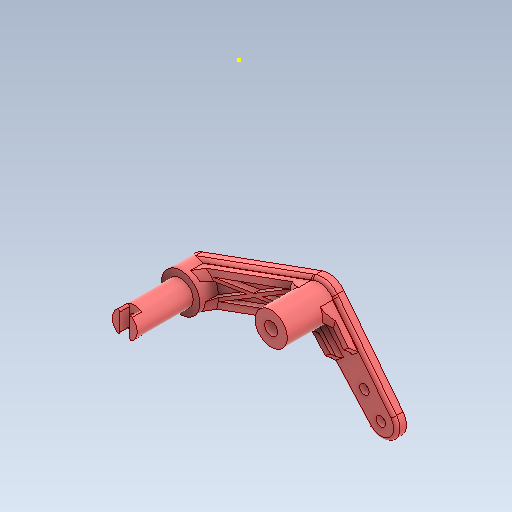
# Autodesk Inventor part: РычагОпорного
Saved by Autodesk Inventor 2020 (Build 240168000, 168)
## iProperties
Created: 2021-03-04
Part Number: РычагОпорного
Material: Пластик АБС
Document SubType Name: Modeling
Designer: I_Love_U_Bogdan
Density: 1.06 g/cm^3
Appearance: Гладкий — красный
Author: I_Love_U_Bogdan
Autodesk Inventor part; units mm, degrees
ref_plane "YZ Plane" through (0, 0, 0) normal (1, 0, 0) x (0, 1, 0)
ref_plane "XZ Plane" through (0, 0, 0) normal (0, 1, 0) x (-1, 0, 0)
ref_plane "XY Plane" through (0, 0, 0) normal (0, 0, 1) x (1, 0, 0)
sketch "Эскиз1" plane through (0, 0, 0) normal (0, 0, 1) x (1, 0, 0)
  arc A0 (12.888162, -136.868324) -> (8.919216, -139.740164) centre (9.43816, -136.27885) ccw
  line L0 (65.630259, -98.70533) -> (12.888162, -136.868324)
  arc A1 (69.599205, -95.83349) -> (65.630259, -98.70533) centre (66.149202, -95.244015) ccw
  line L1 (72.61468, -93.65156) -> (69.599205, -95.83349)
  line L2 (74.525657, -81.736041) -> (72.61468, -93.65156)
  arc A2 (78.84072, -74.295729) -> (74.525657, -81.736041) centre (86.374247, -83.636285) ccw
  arc A3 (78.84072, -74.295729) -> (86.631259, -62.29521) centre (64.401461, -56.392998) ccw
  line L3 (16.222884, -53.884997) -> (16.238465, -53.891971)
  line L4 (2.811002, -47.882385) -> (16.222884, -53.884997)
  line L5 (-128.593437, -142.96368) -> (2.811002, -47.882385)
  arc A4 (-128.593437, -142.96368) -> (-138.339207, -175.63158) centre (-112.179504, -165.648097) ccw
  line L6 (-101.16011, -190.130237) -> (-15.58744, -157.472629)
  line L7 (8.919216, -139.740164) -> (-15.58744, -157.472629)
  circle A5 centre (64.401461, -56.392998) radius 9
  circle A6 centre (25.088911, -52.746159) radius 2.05
  circle A7 centre (25.088911, -52.746159) radius 4.05
  circle A8 centre (-12.498794, -66.426965) radius 3
  line L8 (25.088911, -52.746159) -> (-12.498794, -66.426965)
  line L9 (25.088911, -52.746159) -> (17.64149, -52.746159)
  circle A9 centre (-12.498794, -66.426965) radius 6
  circle A10 centre (25.088911, -52.746159) radius 6
  line L10 (23.03679, -47.108003) -> (-14.550914, -60.788809)
  line L11 (20.157105, -60.926256) -> (-10.446673, -72.06512)
  line L12 (25.088911, -52.746159) -> (44.37254, -75.727492)
  circle A11 centre (44.37254, -75.727492) radius 5
  line L13 (48.307765, -72.643014) -> (29.811181, -49.044785)
  line L14 (40.651577, -79.067318) -> (25.588168, -62.284893)
  arc A12 (25.588168, -62.284893) -> (20.157105, -60.926256) centre (21.867205, -65.62472) ccw
  circle A13 centre (44.37254, -75.727492) radius 1.5
  circle A14 centre (5.904074, -79.867828) radius 1.5
  circle A15 centre (-49.538904, -115.038192) radius 1.5
  circle A16 centre (-106.249947, -156.073027) radius 1.5
  circle A17 centre (-95.647387, -163.91054) radius 1.5
  circle A18 centre (-104.981882, -150.208556) radius 1.5
  circle A19 centre (-50.806969, -120.902663) radius 1.5
  circle A20 centre (7.172139, -74.003358) radius 1.5
  circle A21 centre (44.37254, -75.727492) radius 1.5
  circle A22 centre (-38.936344, -122.875706) radius 1.5
  circle A23 centre (4.636009, -85.732299) radius 1.5
  circle A24 centre (-48.270839, -109.173722) radius 1.5
  circle A25 centre (-107.518011, -161.937497) radius 1.5
  circle A26 centre (-108.786076, -167.801967) radius 1.5
  circle A27 centre (-52.075033, -126.767133) radius 1.5
  circle A28 centre (8.440204, -68.138888) radius 1.5
  circle A29 centre (25.088911, -52.746159) radius 3
  circle A30 centre (-31.622132, -93.780993) radius 3
  circle A31 centre (-88.333174, -134.815827) radius 3
  arc A32 (29.957043, -54.089215) -> (20.651058, -55.156129) centre (25.088911, -52.74616) ccw
  circle A33 centre (60.929555, -78.036608) radius 2.5
  arc A34 (87.361991, -57.739881) -> (86.631259, -62.29521) centre (86.045072, -59.864904) ccw
  arc A35 (87.361991, -57.739881) -> (70.303674, -34.1632) centre (64.401461, -56.392998) ccw
  arc A36 (65.748345, -33.432468) -> (70.303674, -34.1632) centre (67.873368, -34.749387) ccw
  arc A37 (65.748345, -33.432468) -> (47.70038, -40.579273) centre (64.401461, -56.392998) ccw
  spline S0 degree 3 poles (18.301215, -54.651331) (18.607141, -54.740898) (18.915645, -54.821457) (19.697978, -55.001604) (20.173096, -55.089111) (20.651058, -55.156129) knots 0 0 0 0 0.3973381 0.3973381 1 1 1 1
  circle A38 centre (42.757851, -52.921091) radius 2.5
  circle A39 centre (-127.909048, -153.437003) radius 1.5
  circle A40 centre (-114.085694, -155.653954) radius 1.5
  circle A41 centre (-128.700816, -158.373916) radius 1.5
  circle A42 centre (-114.877462, -160.590866) radius 1.5
  circle A43 centre (39.230239, -69.599137) radius 1.5
  spline S1 degree 3 poles (46.97987, -41.376735) (47.210603, -41.109043) (47.447507, -40.84667) (47.69033, -40.589894) (47.693679, -40.586353) (47.697029, -40.582812) (47.70038, -40.579273) knots 0 0 0 0 0.9863956 0.9863956 0.9863956 1 1 1 1 weights 1 1 1 1 1 1 1
  spline S2 degree 3 poles (32.12294, -53.220444) (32.637934, -52.987666) (33.143139, -52.740791) (33.639935, -52.481259) (34.9345, -51.804963) (36.170298, -51.045197) (38.575936, -49.37654) (39.737921, -48.471371) (43.089087, -45.609399) (45.144174, -43.506476) (46.97987, -41.376735) knots 1.47381002 1.47381002 1.47381002 1.47381002 1.63021034 1.63021034 1.63021034 2.03776293 2.03776293 2.44531551 2.44531551 3.26042069 3.26042069 3.26042069 3.26042069 weights 1 1 1 1 1 1 1 1 1 1 1
  spline S3 degree 3 poles (16.238465, -53.891971) (16.912175, -54.193496) (17.601075, -54.446349) (18.301215, -54.651331) knots 0 0 0 0 1 1 1 1 weights 1 1 1 1
  spline S4 degree 3 poles (29.957043, -54.089215) (30.690702, -53.832546) (31.413252, -53.541224) (32.12294, -53.220444) knots 0 0 0 0 1 1 1 1
  line L15 (-130.678918, -195.703821) -> (-138.339207, -175.63158)
  line L16 (-114.628069, -198.278011) -> (-130.678918, -195.703821)
  line L17 (-114.628069, -198.278011) -> (-109.882275, -194.844061)
  line L18 (-101.16011, -190.130237) -> (-109.882275, -194.844061)
  line L19 (8.440204, -68.138888) -> (20.109851, -84.266596)
  line L20 (8.440204, -68.138888) -> (7.172139, -74.003358)
  point P0 (0, 0)
  point P1 (27.141032, -58.384315)
  point P2 (20.623756, -56.75395)
  point P3 (35, -229.746096)
  dimension "d0" = 17
  dimension "d2" = 4.1
  dimension "d3" = 2
  dimension "d4" = 6
  dimension "d5" = 20
  dimension "d6" = 40
  dimension "d7" = 3
  dimension "d8" = 12
  dimension "d9" = 110
  dimension "d10" = 30
  dimension "d11" = 10
  dimension "d12" = 5
  dimension "d22" = 3
  dimension "d54" = 8
  dimension "d87" = 90
  constraints: 18 end point, 10 point on circle, 10 tangent, 9 centre point, 3 coincident, 2 point on line, 1 horizontal, 3 other
  measures "d0" distance from line of L5 L8.start
  measures "d2" diameter of A6
  measures "d3" radial gap between concentric circles of A6 A7
  measures "d4" diameter of A8
  measures "d5" angle of L8 L9
  measures "d6" distance of L8.start L8.end
  measures "d7" radial gap between concentric circles of A8 A9
  measures "d8" diameter of A10
  measures "d9" angle of L8 L12
  measures "d10" distance of L12.start L12.end
  measures "d11" diameter of A11
  measures "d12" radius of A12
  measures "d22" diameter of A13
  measures "d54" distance of A13.centre A43.centre
  measures "d87" angle of L5 L19
extrude "Выдавливание1" add sketch "Эскиз1" along normal blind 3 contours L10 A10 L8 S0 S3 L3 L4 | L4 L3 S3 S0 L8 A9 L10 | A10 S4 A32 L9 | A9 | L13 S2 S4 A10 | L9 A32 L8 A10 | A9 L8 S0 A10 L12 A43 A11 L14 A12 L11 | L13 A11 L12 A43 A10 S4 S2 | A32 S4 A10 L12 A7 L9 | L9 A7 L8 A32 | A10 S0 L8 | L8 A32 S0 A10 | A11 | L9 A29 L8 A7 | A7 L12 A29 L9 | L8 A7 L12 A10 S0 A32 | L8 A29 L12 A7 | A29 L12 A6 L9 | L9 A6 L8 A29 | L8 A6 L12 A29
sketch "Эскиз2" plane through (0, 0, 3) normal (0, 0, 1) x (1, 0, 0)
  arc A0 (27.138911, -52.746159) -> (27.138911, -52.746159) centre (25.088911, -52.746159) ccw
  circle A1 centre (25.088911, -52.746159) radius 5.05
  arc A2 (27.138911, -52.746159) -> (27.138911, -52.746159) centre (25.088911, -52.746159) ccw
  circle A3 centre (25.088911, -52.746159) radius 2.05
  point P0 (0, 0)
  dimension "d28" = 3
  constraints: 2 centre point, 2 coincident
  measures "d28" radial gap between concentric circles of A1 A2
extrude "Выдавливание2" add sketch "Эскиз2" along normal blind 15
sketch "Эскиз3" plane through (0, 0, 3) normal (0, 0, 1) x (1, 0, 0)
  circle A0 centre (-12.498794, -66.426965) radius 3
  circle A1 centre (-12.498794, -66.426965) radius 6
  circle A2 centre (-12.498794, -66.426965) radius 3
  point P0 (0, 0)
  constraints: 1 centre point, 1 coincident
extrude "Выдавливание3" add sketch "Эскиз3" along normal blind 5.7
sketch "Эскиз4" plane through (-12.498794, -66.426965, 8.7) normal (0, 0, 1) x (1, 0, 0)
  circle A0 centre (0, 0) radius 1.5
  circle A1 centre (0, 0) radius 6 projected
  circle A2 centre (0, 0) radius 3 projected
  point P0 (12.498794, 66.426965)
  dimension "d34" = 3
  constraints: 1 centre point
  measures "d34" diameter of A0
extrude "Выдавливание4" add sketch "Эскиз4" against normal blind 3 contours A2
chamfer "Фаска2" distance 1 angle 45 1 edges at (-13.9988, -66.427, 5.7)
sketch "Эскиз5" plane through (-12.498794, -66.426965, 8.7) normal (0, 0, 1) x (1, 0, 0)
  circle A0 centre (0, 0) radius 1.5 projected
  circle A1 centre (0, 0) radius 3.9
  point P0 (12.498794, 66.426965)
  dimension "d40" = 7.8
  constraints: 1 centre point, 1 coincident
  measures "d40" diameter of A1
extrude "Выдавливание5" add sketch "Эскиз5" along normal blind 17.5
sketch "Эскиз6" plane through (-12.498794, -66.426965, 26.2) normal (0, 0, 1) x (1, 0, 0)
  line L0 (-1.5, 5.875938) -> (1.5, 5.875938)
  line L1 (1.5, 5.875938) -> (1.5, -5.875938)
  line L2 (1.5, -5.875938) -> (-1.5, -5.875938)
  line L3 (-1.5, -5.875938) -> (-1.5, 5.875938)
  line L4 (-1.5, 5.875938) -> (1.5, -5.875938) construction
  line L5 (1.5, 5.875938) -> (-1.5, -5.875938) construction
  circle A0 centre (0, 0) radius 1.5
  point P0 (12.498794, 66.426965)
  point P1 (-1.5, 0)
  point P2 (1.5, 0)
  dimension "d43" = 3
  dimension "d44" = 0
  dimension "d45" = 0
  constraints: 12 end point, 2 midpoint, 2 parallel, 1 horizontal, 1 perpendicular
  measures "d43" distance of L1.end L2.end
  measures "d44" distance of A0.centre point (0, 0)
  measures "d45" distance of A0.centre point (0, 0)
extrude "Выдавливание6" cut sketch "Эскиз6" against normal blind 3 contours L0 L1 A0 L3 | A0 L1 L2 L3
fillet "Сопряжение2" radius 0.5 4 edges at (-10.9988, -70.027, 24.7) (-13.9988, -70.027, 24.7) (-13.9988, -62.827, 24.7) (-10.9988, -62.827, 24.7)
chamfer "Фаска4" distance 1 angle 45 2 edges at (37.7302, -69.5991, 0) (42.8725, -75.7275, 0)
sketch "Эскиз9" plane through (0, 0, 3) normal (0, 0, 1) x (1, 0, 0)
  line L0 (-10.446673, -72.06512) -> (20.157105, -60.926256)
  arc A0 (25.588168, -62.284893) -> (20.157105, -60.926256) centre (21.867205, -65.62472) ccw
  line L1 (25.588168, -62.284893) -> (40.651577, -79.067318)
  arc A1 (40.651577, -79.067318) -> (48.307765, -72.643014) centre (44.37254, -75.727492) ccw
  line L2 (48.307765, -72.643014) -> (29.811181, -49.044785)
  arc A2 (29.811181, -49.044785) -> (23.03679, -47.108003) centre (25.088911, -52.746159) ccw
  line L3 (23.03679, -47.108003) -> (-14.550914, -60.788809)
  circle A3 centre (25.088911, -52.746159) radius 5.05
  circle A4 centre (39.230239, -69.599137) radius 1.5
  circle A5 centre (44.37254, -75.727492) radius 1.5
  line L4 (23.624499, -58.60005) -> (-7.672085, -69.991075)
  line L5 (-11.092286, -60.594149) -> (23.378811, -48.047696)
  arc A6 (29.024136, -49.661681) -> (23.378811, -48.047696) centre (25.088911, -52.746159) ccw
  line L6 (29.024136, -49.661681) -> (47.52072, -73.25991)
  arc A7 (41.39577, -78.399353) -> (47.52072, -73.25991) centre (44.37254, -75.727492) ccw
  line L7 (41.39577, -78.399353) -> (23.624499, -58.60005)
  line L8 (25.569827, -57.773208) -> (42.884155, -77.063423)
  arc A8 (42.884155, -77.063423) -> (45.94663, -74.493701) centre (44.37254, -75.727492) ccw
  line L9 (45.94663, -74.493701) -> (27.450046, -50.895472)
  arc A9 (27.450046, -50.895472) -> (24.062851, -49.927081) centre (25.088911, -52.746159) ccw
  line L10 (22.297633, -56.954634) -> (-8.642068, -61.830698) construction
  arc A10 (-10.446673, -72.06512) -> (-14.550914, -60.788809) centre (-12.498794, -66.426965) ccw
  line L11 (-6.589947, -67.468854) -> (20.245512, -51.316479) construction
  circle A11 centre (25.088911, -52.746159) radius 5.05
  line L12 (20.30408, -51.295162) -> (20.245512, -51.316479)
  line L13 (22.219794, -56.46073) -> (9.280504, -58.499949)
  line L14 (6.653546, -58.913955) -> (-6.189347, -60.937981)
  line L15 (-4.137226, -66.576136) -> (7.002019, -59.871378)
  line L16 (9.280504, -58.499949) -> (20.50336, -51.744865)
  line L17 (-8.564229, -62.324602) -> (4.375061, -60.285384)
  line L18 (7.002019, -59.871378) -> (19.844912, -57.847352)
  line L19 (17.792791, -52.209196) -> (6.653546, -58.913955)
  line L20 (4.375061, -60.285384) -> (-6.847794, -67.040468)
  line L21 (17.792791, -52.209196) -> (-6.189347, -60.937981)
  line L22 (-4.137226, -66.576136) -> (19.844912, -57.847352)
  arc A12 (-10.446673, -72.06512) -> (-14.550914, -60.788809) centre (-12.498794, -66.426965) ccw
  line L23 (36.276183, -58.913955) -> (29.014817, -64.605503)
  circle A13 centre (25.088911, -52.746159) radius 2.05
  line L24 (25.088911, -52.746159) -> (32.340958, -61.998432)
  point P0 (0, 0)
  point P1 (6.827783, -59.392666)
  point P2 (6.827783, -59.392666)
  point P3 (21.749924, -56.534782)
  point P4 (20.095819, -51.990166)
  point P5 (22.712688, -48.290144)
  point P6 (29.461436, -50.219595)
  point P7 (29.956078, -54.092706)
  point P8 (-8.178177, -62.263761)
  point P9 (-6.512953, -66.838925)
  point P10 (34.702093, -60.147746)
  point P11 (30.592412, -63.368964)
  dimension "d72" = 1
  constraints: 46 end point, 14 point on circle, 8 parallel, 4 centre point, 3 point on line, 2 midpoint, 2 perpendicular, 4 other
  measures "d72" distance between parallel lines of L0 L4
extrude "Выдавливание8" add sketch "Эскиз9" along normal blind 2 contours A10 L20 L17 L5 A3 L16 L13 L8 L23 L7 L4 | L23 L9 A3 L6
chamfer "Фаска6" distance 2 angle 45 2 edges at (29.8036, -63.9872, 3) (35.4891, -59.5309, 3)
fillet "Сопряжение4" radius 0.99 7 edges at (47.5865, -79.5577, 3) (39.0595, -60.8439, 3) (26.7382, -46.9773, 3) (4.2429, -53.9484, 3) (23.0806, -60.7742, 3) (4.8552, -66.4957, 3) (33.1199, -70.6761, 3)
fillet "Сопряжение5" radius 1 6 edges at (26.9891, -62.3486, 3) (32.9459, -57.9072, 3) (28.7505, -61.3169, 3) (33.4857, -55.3538, 3) (5.8102, -54.4421, 3) (7.9762, -64.2956, 3)
chamfer "Фаска7" distance 2 angle 45 6 edges at (-6.8675, -68.4978, 5) (-9.516, -61.2209, 5) (20.9659, -49.8301, 5) (23.5315, -57.55, 5) (29.9666, -51.4383, 5) (30.093, -53.4256, 5)
sketch "Эскиз10" plane through (0, 0, 3) normal (0, 0, 1) x (1, 0, 0)
  point P0 (0, 0)
